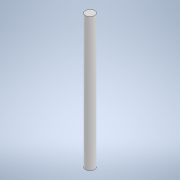
# Autodesk Inventor part: wał_uzębienia
Saved by Autodesk Inventor 2020 (Build 240168000, 168)
## iProperties
Created: 2020-08-10
Part Number: wał_uzębienia
Material: Generic
Document SubType Name: Modeling
Designer: Hesekiel
Density: 1 g/cm^3
Appearance: Default
Author: Hesekiel
Autodesk Inventor part; units mm, degrees
ref_plane "XZ Plane" through (0, 0, 0) normal (0, 1, 0) x (-1, 0, 0)
ref_plane "XY Plane" through (0, 0, 0) normal (0, 0, 1) x (1, 0, 0)
sketch "Sketch1" plane through (0, 0, 0) normal (0, 1, 0) x (-1, 0, 0)
  circle A0 centre (0, 0) radius 7.5
  dimension "d0" = 15
  constraints: 1 centre point, 1 coincident
  measures "d0" diameter of A0
extrude "Extrusion1" add sketch "Sketch1" along normal blind 100
ref_plane "Work Plane1" through (0, 72.5, 0) normal (0, 1, 0) x (1, 0, 0)
sketch "Sketch2" plane through (0, 72.5, 0) normal (0, 1, 0) x (1, 0, 0)
  circle A0 centre (0, 0) radius 7.5 projected
ref_plane "Work Plane2" through (-7.5, 0, 0) normal (1, 0, 0) x (0, 1, 0)
ref_plane "Work Plane3" through (0, 27.5, 0) normal (0, -1, 0) x (1, 0, 0)
sketch "Sketch3" plane through (-7.5, 0, 0) normal (1, 0, 0) x (0, 1, 0)
  line L0 (27.5, -21) -> (27.5, 21) projected
  line L1 (72.5, 21) -> (72.5, -21) projected
  circle A0 centre (27.5, 0) radius 3
  circle A1 centre (72.5, 0) radius 3
  circle A2 centre (27.5, 0) radius 0.75
  circle A3 centre (72.5, 0) radius 0.75
  line L2 (0, -7.5) -> (0, 7.5) projected
  line L3 (27.5, -3) -> (0, -3)
  line L4 (0, -3) -> (0, 3)
  line L5 (0, 3) -> (27.5, 3)
  line L6 (27.5, 3) -> (27.5, -3)
  line L7 (100, -7.5) -> (100, 7.5) projected
  line L8 (72.5, -3) -> (100, -3)
  line L9 (100, -3) -> (100, 3)
  line L10 (100, 3) -> (72.5, 3)
  line L11 (72.5, 3) -> (72.5, -3)
  circle A4 centre (0, 0) radius 3
  line L12 (27.5, -3) -> (72.5, -3)
  line L13 (72.5, -3) -> (72.5, 3)
  line L14 (72.5, 3) -> (27.5, 3)
  line L15 (27.5, 3) -> (27.5, -3)
  point P0 (72.5, 3)
  point P1 (27.5, 3)
  point P2 (72.5, 3)
  point P3 (27.5, 3)
  point P4 (72.5, -3)
  dimension "d5" = 6
  dimension "d6" = 6
  dimension "d7" = 1.5
  dimension "d8" = 1.5
  constraints: 24 end point, 6 parallel, 5 point on line, 3 coincident, 3 horizontal, 3 perpendicular, 2 centre point, 2 midpoint, 9 other
  measures "d7" diameter of A2
  measures "d8" diameter of A3
extrude "Extrusion2" cut sketch "Sketch3" along normal blind 1 contours A2 L0 | L0 A2 | A3 L1 | L1 A3
extrude "Extrusion3" cut sketch "Sketch3" along normal blind 0.5 contours A0 L0 A2 | L0 A2 A0 | A0 L14 A1 L12 | A1 L1 A3 | L1 A3 A1 | A1 L10 L7 L8
chamfer "Chamfer1" distance 0.5 angle 45 1 edges at (-7, 26.75, 0)
chamfer "Chamfer2" distance 0.5 angle 45 1 edges at (-7, 71.75, 0)
sketch "Sketch4" plane through (0, 0, 0) normal (0, -1, 0) x (1, 0, 0)
  circle A0 centre (0, 0) radius 7.5 projected
  circle A1 centre (0, 0) radius 7.5
  constraints: 1 centre point, 1 coincident
extrude "Extrusion4" add sketch "Sketch4" along normal blind 60
sketch "Sketch5" plane through (0, 100, 0) normal (0, 1, 0) x (1, 0, 0)
  arc A0 (-7, -2.6926) -> (-7, 2.6926) centre (0, 0) ccw projected
  line L0 (-7, 2.6926) -> (-7, -2.6926) projected
  arc A1 (-7, -2.6926) -> (-7, 2.6926) centre (0, 0) ccw projected
  point P0 (-7, 2.6926)
extrude "Extrusion5" add sketch "Sketch5" along normal blind 60
body "Solid1"
